Autodesk Inventor part; units mm, degrees
(part 2 of 3)
sketch "スケッチ2" plane through (0, 0, 3) normal (0, 0, 1) x (1, 0, 0)
  line L0 (168.378, 87.7618) -> (167.765, 88.2934) projected
  arc A0 (167.765, 88.2934) -> (169.0746, 89.9356) centre (148.5, 105) ccw projected
  line L1 (169.0746, 89.9356) -> (169.7292, 89.4562) projected
  arc A1 (169.7292, 89.4562) -> (170.0536, 89.2707) centre (171.1243, 91.5187) ccw projected
  arc A2 (170.0536, 89.2707) -> (171.1838, 88.8403) centre (173.0427, 95.4208) ccw projected
  arc A3 (171.1838, 88.8403) -> (173.5053, 88.4249) centre (174.4109, 100.1798) ccw projected
  arc A4 (173.5053, 88.4249) -> (174.2831, 89.6627) centre (148.5, 105) ccw projected
  arc A5 (174.2831, 89.6627) -> (172.9015, 91.5741) centre (164.0852, 83.7465) ccw projected
  arc A6 (172.9015, 91.5741) -> (172.0234, 92.4056) centre (167.7792, 87.0441) ccw projected
  arc A7 (172.0234, 92.4056) -> (171.7155, 92.6173) centre (170.4625, 90.4655) ccw projected
  line L2 (171.7155, 92.6173) -> (170.9996, 92.9992) projected
  arc A8 (170.9996, 92.9992) -> (171.9109, 94.8915) centre (148.5, 105) ccw projected
  line L3 (171.9109, 94.8915) -> (172.6558, 94.5699) projected
  arc A9 (172.6558, 94.5699) -> (173.0133, 94.4612) centre (173.5569, 96.8911) ccw projected
  arc A10 (173.0133, 94.4612) -> (174.2109, 94.2931) centre (174.5589, 101.1222) ccw projected
  arc A11 (174.2109, 94.2931) -> (176.5667, 94.4046) centre (174.8339, 106.0664) ccw projected
  arc A12 (176.5667, 94.4046) -> (177.0495, 95.7845) centre (148.5, 105) ccw projected
  arc A13 (177.0495, 95.7845) -> (175.2773, 97.3405) centre (168.4238, 87.7474) ccw projected
  arc A14 (175.2773, 97.3405) -> (174.2362, 97.9558) centre (171.2914, 91.7843) ccw projected
  arc A15 (174.2362, 97.9558) -> (173.8888, 98.0937) centre (173.1461, 95.717) ccw projected
  line L4 (173.8888, 98.0937) -> (173.1059, 98.3067) projected
  arc A16 (173.1059, 98.3067) -> (173.5733, 100.3544) centre (148.5, 105) ccw projected
  line L5 (173.5733, 100.3544) -> (174.3711, 100.2066) projected
  arc A17 (174.3711, 100.2066) -> (174.7439, 100.1801) centre (174.7331, 102.6701) ccw projected
  arc A18 (174.7439, 100.1801) -> (175.9488, 100.2827) centre (174.7684, 107.0181) ccw projected
  arc A19 (175.9488, 100.2827) -> (178.2207, 100.9157) centre (173.9363, 111.8995) ccw projected
  arc A20 (178.2207, 100.9157) -> (178.3844, 102.3684) centre (148.5, 105) ccw projected
  arc A21 (178.3844, 102.3684) -> (176.3103, 103.4911) centre (171.7633, 92.6134) ccw projected
  arc A22 (176.3103, 103.4911) -> (175.1584, 103.8592) centre (173.6608, 97.1872) ccw projected
  arc A23 (175.1584, 103.8592) -> (174.7891, 103.9164) centre (174.5938, 101.4341) ccw projected
  line L6 (174.7891, 103.9164) -> (173.9784, 103.9498) projected
  arc A24 (173.9784, 103.9498) -> (173.9784, 106.0502) centre (148.5, 105) ccw projected
  line L7 (173.9784, 106.0502) -> (174.7891, 106.0836) projected
  arc A25 (174.7891, 106.0836) -> (175.1584, 106.1408) centre (174.5938, 108.5659) ccw projected
  arc A26 (175.1584, 106.1408) -> (176.3103, 106.5089) centre (173.6608, 112.8128) ccw projected
  arc A27 (176.3103, 106.5089) -> (178.3844, 107.6316) centre (171.7633, 117.3866) ccw projected
  arc A28 (178.3844, 107.6316) -> (178.2207, 109.0843) centre (148.5, 105) ccw projected
  arc A29 (178.2207, 109.0843) -> (175.9488, 109.7173) centre (173.9363, 98.1005) ccw projected
  arc A30 (175.9488, 109.7173) -> (174.7439, 109.8199) centre (174.7684, 102.9819) ccw projected
  arc A31 (174.7439, 109.8199) -> (174.3711, 109.7934) centre (174.7331, 107.3299) ccw projected
  line L8 (174.3711, 109.7934) -> (173.5733, 109.6456) projected
  arc A32 (173.5733, 109.6456) -> (173.1059, 111.6933) centre (148.5, 105) ccw projected
  line L9 (173.1059, 111.6933) -> (173.8888, 111.9063) projected
  arc A33 (173.8888, 111.9063) -> (174.2362, 112.0442) centre (173.1461, 114.283) ccw projected
  arc A34 (174.2362, 112.0442) -> (175.2773, 112.6595) centre (171.2914, 118.2157) ccw projected
  arc A35 (175.2773, 112.6595) -> (177.0495, 114.2155) centre (168.4238, 122.2526) ccw projected
  arc A36 (177.0495, 114.2155) -> (176.5667, 115.5954) centre (148.5, 105) ccw projected
  arc A37 (176.5667, 115.5954) -> (174.2109, 115.7069) centre (174.8339, 103.9336) ccw projected
  arc A38 (174.2109, 115.7069) -> (173.0133, 115.5388) centre (174.5589, 108.8778) ccw projected
  arc A39 (173.0133, 115.5388) -> (172.6558, 115.4301) centre (173.5569, 113.1089) ccw projected
  line L10 (172.6558, 115.4301) -> (171.9109, 115.1085) projected
  arc A40 (171.9109, 115.1085) -> (170.9996, 117.0008) centre (148.5, 105) ccw projected
  line L11 (170.9996, 117.0008) -> (171.7155, 117.3827) projected
  arc A41 (171.7155, 117.3827) -> (172.0234, 117.5944) centre (170.4625, 119.5345) ccw projected
  arc A42 (172.0234, 117.5944) -> (172.9015, 118.4259) centre (167.7792, 122.9559) ccw projected
  arc A43 (172.9015, 118.4259) -> (174.2831, 120.3373) centre (164.0852, 126.2535) ccw projected
  arc A44 (174.2831, 120.3373) -> (173.5053, 121.5751) centre (148.5, 105) ccw projected
  arc A45 (173.5053, 121.5751) -> (171.1838, 121.1597) centre (174.4109, 109.8202) ccw projected
  arc A46 (171.1838, 121.1597) -> (170.0536, 120.7293) centre (173.0427, 114.5792) ccw projected
  arc A47 (170.0536, 120.7293) -> (169.7292, 120.5438) centre (171.1243, 118.4813) ccw projected
  line L12 (169.7292, 120.5438) -> (169.0746, 120.0644) projected
  arc A48 (169.0746, 120.0644) -> (167.765, 121.7066) centre (148.5, 105) ccw projected
  line L13 (167.765, 121.7066) -> (168.378, 122.2382) projected
  arc A49 (168.378, 122.2382) -> (168.6311, 122.5131) centre (166.6776, 124.0572) ccw projected
  arc A50 (168.6311, 122.5131) -> (169.3022, 123.5192) centre (163.3003, 126.7958) ccw projected
  arc A51 (169.3022, 123.5192) -> (170.2238, 125.69) centre (158.9651, 129.1887) ccw projected
  arc A52 (170.2238, 125.69) -> (169.19, 126.7238) centre (148.5, 105) ccw projected
  arc A53 (169.19, 126.7238) -> (167.0192, 125.8022) centre (172.6887, 115.4651) ccw projected
  arc A54 (167.0192, 125.8022) -> (166.0131, 125.1311) centre (170.2958, 119.8003) ccw projected
  arc A55 (166.0131, 125.1311) -> (165.7382, 124.878) centre (167.5572, 123.1776) ccw projected
  line L14 (165.7382, 124.878) -> (165.2066, 124.265) projected
  arc A56 (165.2066, 124.265) -> (163.5644, 125.5746) centre (148.5, 105) ccw projected
  line L15 (163.5644, 125.5746) -> (164.0438, 126.2292) projected
  arc A57 (164.0438, 126.2292) -> (164.2293, 126.5536) centre (161.9813, 127.6243) ccw projected
  arc A58 (164.2293, 126.5536) -> (164.6597, 127.6838) centre (158.0792, 129.5427) ccw projected
  arc A59 (164.6597, 127.6838) -> (165.0751, 130.0053) centre (153.3202, 130.9109) ccw projected
  arc A60 (165.0751, 130.0053) -> (163.8373, 130.7831) centre (148.5, 105) ccw projected
  arc A61 (163.8373, 130.7831) -> (161.9259, 129.4015) centre (169.7535, 120.5852) ccw projected
  arc A62 (161.9259, 129.4015) -> (161.0944, 128.5234) centre (166.4559, 124.2792) ccw projected
  arc A63 (161.0944, 128.5234) -> (160.8827, 128.2155) centre (163.0345, 126.9625) ccw projected
  line L16 (160.8827, 128.2155) -> (160.5008, 127.4996) projected
  arc A64 (160.5008, 127.4996) -> (158.6085, 128.4109) centre (148.5, 105) ccw projected
  line L17 (158.6085, 128.4109) -> (158.9301, 129.1558) projected
  arc A65 (158.9301, 129.1558) -> (159.0388, 129.5133) centre (156.6089, 130.0569) ccw projected
  arc A66 (159.0388, 129.5133) -> (159.2069, 130.7109) centre (152.3778, 131.0589) ccw projected
  arc A67 (159.2069, 130.7109) -> (159.0954, 133.0667) centre (147.4336, 131.3339) ccw projected
  arc A68 (159.0954, 133.0667) -> (157.7155, 133.5495) centre (148.5, 105) ccw projected
  arc A69 (157.7155, 133.5495) -> (156.1595, 131.7773) centre (165.7526, 124.9238) ccw projected
  arc A70 (156.1595, 131.7773) -> (155.5442, 130.7362) centre (161.7157, 127.7914) ccw projected
  arc A71 (155.5442, 130.7362) -> (155.4063, 130.3888) centre (157.783, 129.6461) ccw projected
  line L18 (155.4063, 130.3888) -> (155.1933, 129.6059) projected
  arc A72 (155.1933, 129.6059) -> (153.1456, 130.0733) centre (148.5, 105) ccw projected
  line L19 (153.1456, 130.0733) -> (153.2934, 130.8711) projected
  arc A73 (153.2934, 130.8711) -> (153.3199, 131.2439) centre (150.8299, 131.2331) ccw projected
  arc A74 (153.3199, 131.2439) -> (153.2173, 132.4488) centre (146.4819, 131.2684) ccw projected
  arc A75 (153.2173, 132.4488) -> (152.5843, 134.7207) centre (141.6005, 130.4363) ccw projected
  arc A76 (152.5843, 134.7207) -> (151.1316, 134.8844) centre (148.5, 105) ccw projected
  arc A77 (151.1316, 134.8844) -> (150.0089, 132.8103) centre (160.8866, 128.2633) ccw projected
  arc A78 (150.0089, 132.8103) -> (149.6408, 131.6584) centre (156.3128, 130.1608) ccw projected
  arc A79 (149.6408, 131.6584) -> (149.5836, 131.2891) centre (152.0659, 131.0938) ccw projected
  line L20 (149.5836, 131.2891) -> (149.5502, 130.4784) projected
  arc A80 (149.5502, 130.4784) -> (147.4498, 130.4784) centre (148.5, 105) ccw projected
  line L21 (147.4498, 130.4784) -> (147.4164, 131.2891) projected
  arc A81 (147.4164, 131.2891) -> (147.3592, 131.6584) centre (144.9341, 131.0938) ccw projected
  arc A82 (147.3592, 131.6584) -> (146.9911, 132.8103) centre (140.6872, 130.1608) ccw projected
  arc A83 (146.9911, 132.8103) -> (145.8684, 134.8844) centre (136.1134, 128.2633) ccw projected
  arc A84 (145.8684, 134.8844) -> (144.4157, 134.7207) centre (148.5, 105) ccw projected
  arc A85 (144.4157, 134.7207) -> (143.7827, 132.4488) centre (155.3995, 130.4363) ccw projected
  arc A86 (143.7827, 132.4488) -> (143.6801, 131.2439) centre (150.5181, 131.2684) ccw projected
  arc A87 (143.6801, 131.2439) -> (143.7066, 130.8711) centre (146.1701, 131.2331) ccw projected
  line L22 (143.7066, 130.8711) -> (143.8544, 130.0733) projected
  arc A88 (143.8544, 130.0733) -> (141.8067, 129.6059) centre (148.5, 105) ccw projected
  line L23 (141.8067, 129.6059) -> (141.5937, 130.3888) projected
  arc A89 (141.5937, 130.3888) -> (141.4558, 130.7362) centre (139.217, 129.6461) ccw projected
  arc A90 (141.4558, 130.7362) -> (140.8405, 131.7773) centre (135.2843, 127.7914) ccw projected
  arc A91 (140.8405, 131.7773) -> (139.2845, 133.5495) centre (131.2474, 124.9238) ccw projected
  arc A92 (139.2845, 133.5495) -> (137.9046, 133.0667) centre (148.5, 105) ccw projected
  arc A93 (137.9046, 133.0667) -> (137.7931, 130.7109) centre (149.5664, 131.3339) ccw projected
  arc A94 (137.7931, 130.7109) -> (137.9612, 129.5133) centre (144.6222, 131.0589) ccw projected
  arc A95 (137.9612, 129.5133) -> (138.0699, 129.1558) centre (140.3911, 130.0569) ccw projected
  line L24 (138.0699, 129.1558) -> (138.3915, 128.4109) projected
  arc A96 (138.3915, 128.4109) -> (136.4992, 127.4996) centre (148.5, 105) ccw projected
  line L25 (136.4992, 127.4996) -> (136.1173, 128.2155) projected
  arc A97 (136.1173, 128.2155) -> (135.9056, 128.5234) centre (133.9655, 126.9625) ccw projected
  arc A98 (135.9056, 128.5234) -> (135.0741, 129.4015) centre (130.5441, 124.2792) ccw projected
  arc A99 (135.0741, 129.4015) -> (133.1627, 130.7831) centre (127.2465, 120.5852) ccw projected
  arc A100 (133.1627, 130.7831) -> (131.9249, 130.0053) centre (148.5, 105) ccw projected
  arc A101 (131.9249, 130.0053) -> (132.3403, 127.6838) centre (143.6798, 130.9109) ccw projected
  arc A102 (132.3403, 127.6838) -> (132.7707, 126.5536) centre (138.9208, 129.5427) ccw projected
  arc A103 (132.7707, 126.5536) -> (132.9562, 126.2292) centre (135.0187, 127.6243) ccw projected
  line L26 (132.9562, 126.2292) -> (133.4356, 125.5746) projected
  arc A104 (133.4356, 125.5746) -> (131.7934, 124.265) centre (148.5, 105) ccw projected
  line L27 (131.7934, 124.265) -> (131.2618, 124.878) projected
  arc A105 (131.2618, 124.878) -> (130.9869, 125.1311) centre (129.4428, 123.1776) ccw projected
  arc A106 (130.9869, 125.1311) -> (129.9808, 125.8022) centre (126.7042, 119.8003) ccw projected
  arc A107 (129.9808, 125.8022) -> (127.81, 126.7238) centre (124.3113, 115.4651) ccw projected
  arc A108 (127.81, 126.7238) -> (126.7762, 125.69) centre (148.5, 105) ccw projected
  arc A109 (126.7762, 125.69) -> (127.6978, 123.5192) centre (138.0349, 129.1887) ccw projected
  arc A110 (127.6978, 123.5192) -> (128.3689, 122.5131) centre (133.6997, 126.7958) ccw projected
  arc A111 (128.3689, 122.5131) -> (128.622, 122.2382) centre (130.3224, 124.0572) ccw projected
  line L28 (128.622, 122.2382) -> (129.235, 121.7066) projected
  arc A112 (129.235, 121.7066) -> (127.9254, 120.0644) centre (148.5, 105) ccw projected
  line L29 (127.9254, 120.0644) -> (127.2708, 120.5438) projected
  arc A113 (127.2708, 120.5438) -> (126.9464, 120.7293) centre (125.8757, 118.4813) ccw projected
  arc A114 (126.9464, 120.7293) -> (125.8162, 121.1597) centre (123.9573, 114.5792) ccw projected
  arc A115 (125.8162, 121.1597) -> (123.4947, 121.5751) centre (122.5891, 109.8202) ccw projected
  arc A116 (123.4947, 121.5751) -> (122.7169, 120.3373) centre (148.5, 105) ccw projected
  arc A117 (122.7169, 120.3373) -> (124.0985, 118.4259) centre (132.9148, 126.2535) ccw projected
  arc A118 (124.0985, 118.4259) -> (124.9766, 117.5944) centre (129.2208, 122.9559) ccw projected
  arc A119 (124.9766, 117.5944) -> (125.2845, 117.3827) centre (126.5375, 119.5345) ccw projected
  line L30 (125.2845, 117.3827) -> (126.0004, 117.0008) projected
  arc A120 (126.0004, 117.0008) -> (125.0891, 115.1085) centre (148.5, 105) ccw projected
  line L31 (125.0891, 115.1085) -> (124.3442, 115.4301) projected
  arc A121 (124.3442, 115.4301) -> (123.9867, 115.5388) centre (123.4431, 113.1089) ccw projected
  arc A122 (123.9867, 115.5388) -> (122.7891, 115.7069) centre (122.4411, 108.8778) ccw projected
  arc A123 (122.7891, 115.7069) -> (120.4333, 115.5954) centre (122.1661, 103.9336) ccw projected
  arc A124 (120.4333, 115.5954) -> (119.9505, 114.2155) centre (148.5, 105) ccw projected
  arc A125 (119.9505, 114.2155) -> (121.7227, 112.6595) centre (128.5762, 122.2526) ccw projected
  arc A126 (121.7227, 112.6595) -> (122.7638, 112.0442) centre (125.7086, 118.2157) ccw projected
  arc A127 (122.7638, 112.0442) -> (123.1112, 111.9063) centre (123.8539, 114.283) ccw projected
  line L32 (123.1112, 111.9063) -> (123.8941, 111.6933) projected
  arc A128 (123.8941, 111.6933) -> (123.4267, 109.6456) centre (148.5, 105) ccw projected
  line L33 (123.4267, 109.6456) -> (122.6289, 109.7934) projected
  arc A129 (122.6289, 109.7934) -> (122.2561, 109.8199) centre (122.2669, 107.3299) ccw projected
  arc A130 (122.2561, 109.8199) -> (121.0512, 109.7173) centre (122.2316, 102.9819) ccw projected
  arc A131 (121.0512, 109.7173) -> (118.7793, 109.0843) centre (123.0637, 98.1005) ccw projected
  arc A132 (118.7793, 109.0843) -> (118.6156, 107.6316) centre (148.5, 105) ccw projected
  arc A133 (118.6156, 107.6316) -> (120.6897, 106.5089) centre (125.2367, 117.3866) ccw projected
  arc A134 (120.6897, 106.5089) -> (121.8416, 106.1408) centre (123.3392, 112.8128) ccw projected
  arc A135 (121.8416, 106.1408) -> (122.2109, 106.0836) centre (122.4062, 108.5659) ccw projected
  line L34 (122.2109, 106.0836) -> (123.0216, 106.0502) projected
  arc A136 (123.0216, 106.0502) -> (123.0216, 103.9498) centre (148.5, 105) ccw projected
  line L35 (123.0216, 103.9498) -> (122.2109, 103.9164) projected
  arc A137 (122.2109, 103.9164) -> (121.8416, 103.8592) centre (122.4062, 101.4341) ccw projected
  arc A138 (121.8416, 103.8592) -> (120.6897, 103.4911) centre (123.3392, 97.1872) ccw projected
  arc A139 (120.6897, 103.4911) -> (118.6156, 102.3684) centre (125.2367, 92.6134) ccw projected
  arc A140 (118.6156, 102.3684) -> (118.7793, 100.9157) centre (148.5, 105) ccw projected
  arc A141 (118.7793, 100.9157) -> (121.0512, 100.2827) centre (123.0637, 111.8995) ccw projected
  arc A142 (121.0512, 100.2827) -> (122.2561, 100.1801) centre (122.2316, 107.0181) ccw projected
  arc A143 (122.2561, 100.1801) -> (122.6289, 100.2066) centre (122.2669, 102.6701) ccw projected
  line L36 (122.6289, 100.2066) -> (123.4267, 100.3544) projected
  arc A144 (123.4267, 100.3544) -> (123.8941, 98.3067) centre (148.5, 105) ccw projected
  line L37 (123.8941, 98.3067) -> (123.1112, 98.0937) projected
  arc A145 (123.1112, 98.0937) -> (122.7638, 97.9558) centre (123.8539, 95.717) ccw projected
  arc A146 (122.7638, 97.9558) -> (121.7227, 97.3405) centre (125.7086, 91.7843) ccw projected
  arc A147 (121.7227, 97.3405) -> (119.9505, 95.7845) centre (128.5762, 87.7474) ccw projected
  arc A148 (119.9505, 95.7845) -> (120.4333, 94.4046) centre (148.5, 105) ccw projected
  arc A149 (120.4333, 94.4046) -> (122.7891, 94.2931) centre (122.1661, 106.0664) ccw projected
  arc A150 (122.7891, 94.2931) -> (123.9867, 94.4612) centre (122.4411, 101.1222) ccw projected
  arc A151 (123.9867, 94.4612) -> (124.3442, 94.5699) centre (123.4431, 96.8911) ccw projected
  line L38 (124.3442, 94.5699) -> (125.0891, 94.8915) projected
  arc A152 (125.0891, 94.8915) -> (126.0004, 92.9992) centre (148.5, 105) ccw projected
  line L39 (126.0004, 92.9992) -> (125.2845, 92.6173) projected
  arc A153 (125.2845, 92.6173) -> (124.9766, 92.4056) centre (126.5375, 90.4655) ccw projected
  arc A154 (124.9766, 92.4056) -> (124.0985, 91.5741) centre (129.2208, 87.0441) ccw projected
  arc A155 (124.0985, 91.5741) -> (122.7169, 89.6627) centre (132.9148, 83.7465) ccw projected
  arc A156 (122.7169, 89.6627) -> (123.4947, 88.4249) centre (148.5, 105) ccw projected
  arc A157 (123.4947, 88.4249) -> (125.8162, 88.8403) centre (122.5891, 100.1798) ccw projected
  arc A158 (125.8162, 88.8403) -> (126.9464, 89.2707) centre (123.9573, 95.4208) ccw projected
  arc A159 (126.9464, 89.2707) -> (127.2708, 89.4562) centre (125.8757, 91.5187) ccw projected
  line L40 (127.2708, 89.4562) -> (127.9254, 89.9356) projected
  arc A160 (127.9254, 89.9356) -> (129.235, 88.2934) centre (148.5, 105) ccw projected
  line L41 (129.235, 88.2934) -> (128.622, 87.7618) projected
  arc A161 (128.622, 87.7618) -> (128.3689, 87.4869) centre (130.3224, 85.9428) ccw projected
  arc A162 (128.3689, 87.4869) -> (127.6978, 86.4808) centre (133.6997, 83.2042) ccw projected
  arc A163 (127.6978, 86.4808) -> (126.7762, 84.31) centre (138.0349, 80.8113) ccw projected
  arc A164 (126.7762, 84.31) -> (127.81, 83.2762) centre (148.5, 105) ccw projected
  arc A165 (127.81, 83.2762) -> (129.9808, 84.1978) centre (124.3113, 94.5349) ccw projected
  arc A166 (129.9808, 84.1978) -> (130.9869, 84.8689) centre (126.7042, 90.1997) ccw projected
  arc A167 (130.9869, 84.8689) -> (131.2618, 85.122) centre (129.4428, 86.8224) ccw projected
  line L42 (131.2618, 85.122) -> (131.7934, 85.735) projected
  arc A168 (131.7934, 85.735) -> (133.4356, 84.4254) centre (148.5, 105) ccw projected
  line L43 (133.4356, 84.4254) -> (132.9562, 83.7708) projected
  arc A169 (132.9562, 83.7708) -> (132.7707, 83.4464) centre (135.0187, 82.3757) ccw projected
  arc A170 (132.7707, 83.4464) -> (132.3403, 82.3162) centre (138.9208, 80.4573) ccw projected
  arc A171 (132.3403, 82.3162) -> (131.9249, 79.9947) centre (143.6798, 79.0891) ccw projected
  arc A172 (131.9249, 79.9947) -> (133.1627, 79.2169) centre (148.5, 105) ccw projected
  arc A173 (133.1627, 79.2169) -> (135.0741, 80.5985) centre (127.2465, 89.4148) ccw projected
  arc A174 (135.0741, 80.5985) -> (135.9056, 81.4766) centre (130.5441, 85.7208) ccw projected
  arc A175 (135.9056, 81.4766) -> (136.1173, 81.7845) centre (133.9655, 83.0375) ccw projected
  line L44 (136.1173, 81.7845) -> (136.4992, 82.5004) projected
  arc A176 (136.4992, 82.5004) -> (138.3915, 81.5891) centre (148.5, 105) ccw projected
  line L45 (138.3915, 81.5891) -> (138.0699, 80.8442) projected
  arc A177 (138.0699, 80.8442) -> (137.9612, 80.4867) centre (140.3911, 79.9431) ccw projected
  arc A178 (137.9612, 80.4867) -> (137.7931, 79.2891) centre (144.6222, 78.9411) ccw projected
  arc A179 (137.7931, 79.2891) -> (137.9046, 76.9333) centre (149.5664, 78.6661) ccw projected
  arc A180 (137.9046, 76.9333) -> (139.2845, 76.4505) centre (148.5, 105) ccw projected
  arc A181 (139.2845, 76.4505) -> (140.8405, 78.2227) centre (131.2474, 85.0762) ccw projected
  arc A182 (140.8405, 78.2227) -> (141.4558, 79.2638) centre (135.2843, 82.2086) ccw projected
  arc A183 (141.4558, 79.2638) -> (141.5937, 79.6112) centre (139.217, 80.3539) ccw projected
  line L46 (141.5937, 79.6112) -> (141.8067, 80.3941) projected
  arc A184 (141.8067, 80.3941) -> (143.8544, 79.9267) centre (148.5, 105) ccw projected
  line L47 (143.8544, 79.9267) -> (143.7066, 79.1289) projected
  arc A185 (143.7066, 79.1289) -> (143.6801, 78.7561) centre (146.1701, 78.7669) ccw projected
  arc A186 (143.6801, 78.7561) -> (143.7827, 77.5512) centre (150.5181, 78.7316) ccw projected
  arc A187 (143.7827, 77.5512) -> (144.4157, 75.2793) centre (155.3995, 79.5637) ccw projected
  arc A188 (144.4157, 75.2793) -> (145.8684, 75.1156) centre (148.5, 105) ccw projected
  arc A189 (145.8684, 75.1156) -> (146.9911, 77.1897) centre (136.1134, 81.7367) ccw projected
  arc A190 (146.9911, 77.1897) -> (147.3592, 78.3416) centre (140.6872, 79.8392) ccw projected
  arc A191 (147.3592, 78.3416) -> (147.4164, 78.7109) centre (144.9341, 78.9062) ccw projected
  line L48 (147.4164, 78.7109) -> (147.4498, 79.5216) projected
  arc A192 (147.4498, 79.5216) -> (149.5502, 79.5216) centre (148.5, 105) ccw projected
  line L49 (149.5502, 79.5216) -> (149.5836, 78.7109) projected
  arc A193 (149.5836, 78.7109) -> (149.6408, 78.3416) centre (152.0659, 78.9062) ccw projected
  arc A194 (149.6408, 78.3416) -> (150.0089, 77.1897) centre (156.3128, 79.8392) ccw projected
  arc A195 (150.0089, 77.1897) -> (151.1316, 75.1156) centre (160.8866, 81.7367) ccw projected
  arc A196 (151.1316, 75.1156) -> (152.5843, 75.2793) centre (148.5, 105) ccw projected
  arc A197 (152.5843, 75.2793) -> (153.2173, 77.5512) centre (141.6005, 79.5637) ccw projected
  arc A198 (153.2173, 77.5512) -> (153.3199, 78.7561) centre (146.4819, 78.7316) ccw projected
  arc A199 (153.3199, 78.7561) -> (153.2934, 79.1289) centre (150.8299, 78.7669) ccw projected
  line L50 (153.2934, 79.1289) -> (153.1456, 79.9267) projected
  arc A200 (153.1456, 79.9267) -> (155.1933, 80.3941) centre (148.5, 105) ccw projected
  line L51 (155.1933, 80.3941) -> (155.4063, 79.6112) projected
  arc A201 (155.4063, 79.6112) -> (155.5442, 79.2638) centre (157.783, 80.3539) ccw projected
  arc A202 (155.5442, 79.2638) -> (156.1595, 78.2227) centre (161.7157, 82.2086) ccw projected
  arc A203 (156.1595, 78.2227) -> (157.7155, 76.4505) centre (165.7526, 85.0762) ccw projected
  arc A204 (157.7155, 76.4505) -> (159.0954, 76.9333) centre (148.5, 105) ccw projected
  arc A205 (159.0954, 76.9333) -> (159.2069, 79.2891) centre (147.4336, 78.6661) ccw projected
  arc A206 (159.2069, 79.2891) -> (159.0388, 80.4867) centre (152.3778, 78.9411) ccw projected
  arc A207 (159.0388, 80.4867) -> (158.9301, 80.8442) centre (156.6089, 79.9431) ccw projected
  line L52 (158.9301, 80.8442) -> (158.6085, 81.5891) projected
  arc A208 (158.6085, 81.5891) -> (160.5008, 82.5004) centre (148.5, 105) ccw projected
  line L53 (160.5008, 82.5004) -> (160.8827, 81.7845) projected
  arc A209 (160.8827, 81.7845) -> (161.0944, 81.4766) centre (163.0345, 83.0375) ccw projected
  arc A210 (161.0944, 81.4766) -> (161.9259, 80.5985) centre (166.4559, 85.7208) ccw projected
  arc A211 (161.9259, 80.5985) -> (163.8373, 79.2169) centre (169.7535, 89.4148) ccw projected
  arc A212 (163.8373, 79.2169) -> (165.0751, 79.9947) centre (148.5, 105) ccw projected
  arc A213 (165.0751, 79.9947) -> (164.6597, 82.3162) centre (153.3202, 79.0891) ccw projected
  arc A214 (164.6597, 82.3162) -> (164.2293, 83.4464) centre (158.0792, 80.4573) ccw projected
  arc A215 (164.2293, 83.4464) -> (164.0438, 83.7708) centre (161.9813, 82.3757) ccw projected
  line L54 (164.0438, 83.7708) -> (163.5644, 84.4254) projected
  arc A216 (163.5644, 84.4254) -> (165.2066, 85.735) centre (148.5, 105) ccw projected
  line L55 (165.2066, 85.735) -> (165.7382, 85.122) projected
  arc A217 (165.7382, 85.122) -> (166.0131, 84.8689) centre (167.5572, 86.8224) ccw projected
  arc A218 (166.0131, 84.8689) -> (167.0192, 84.1978) centre (170.2958, 90.1997) ccw projected
  arc A219 (167.0192, 84.1978) -> (169.19, 83.2762) centre (172.6887, 94.5349) ccw projected
  arc A220 (169.19, 83.2762) -> (170.2238, 84.31) centre (148.5, 105) ccw projected
  arc A221 (170.2238, 84.31) -> (169.3022, 86.4808) centre (158.9651, 80.8113) ccw projected
  arc A222 (169.3022, 86.4808) -> (168.6311, 87.4869) centre (163.3003, 83.2042) ccw projected
  arc A223 (168.6311, 87.4869) -> (168.378, 87.7618) centre (166.6776, 85.9428) ccw projected
  arc A224 (148.5, 98.8449) -> (147.3388, 98.1857) centre (148.8502, 96.8758) ccw projected
  arc A225 (148.5, 98.8449) -> (148.2359, 98.874) centre (148.1498, 96.8758) ccw projected
  arc A226 (148.2359, 98.874) -> (148.7641, 98.874) centre (148.5, 105) ccw projected
  arc A227 (148.7641, 98.874) -> (148.5, 98.8449) centre (148.8502, 96.8758) ccw projected
  arc A228 (149.6612, 98.1857) -> (148.5, 98.8449) centre (148.1498, 96.8758) ccw projected
  line L56 (149.6612, 98.1857) -> (158.7085, 87.7462) projected
  arc A229 (158.0456, 84.6252) -> (158.7085, 87.7462) centre (157.1971, 86.4363) ccw projected
  arc A230 (138.9544, 84.6252) -> (158.0456, 84.6252) centre (148.5, 105) ccw projected
  arc A231 (138.2915, 87.7462) -> (138.9544, 84.6252) centre (139.8029, 86.4363) ccw projected
  line L57 (138.2915, 87.7462) -> (147.3388, 98.1857) projected
  arc A232 (154.3538, 103.098) -> (154.622, 101.7899) centre (156.3348, 102.8226) ccw projected
  arc A233 (154.3538, 103.098) -> (154.2446, 102.8558) centre (156.1183, 102.1564) ccw projected
  arc A234 (154.2446, 102.8558) -> (154.4078, 103.3581) centre (148.5, 105) ccw projected
  arc A235 (154.4078, 103.3581) -> (154.3538, 103.098) centre (156.3348, 102.8226) ccw projected
  arc A236 (155.3396, 103.9986) -> (154.3538, 103.098) centre (156.1183, 102.1564) ccw projected
  line L58 (155.3396, 103.9986) -> (168.064, 109.3772) projected
  arc A237 (170.8273, 107.7823) -> (168.064, 109.3772) centre (168.8427, 107.535) ccw projected
  arc A238 (164.9278, 89.6254) -> (170.8273, 107.7823) centre (148.5, 105) ccw projected
  arc A239 (161.7547, 89.9594) -> (164.9278, 89.6254) centre (163.4675, 90.992) ccw projected
  line L59 (161.7547, 89.9594) -> (154.622, 101.7899) projected
  arc A240 (142.7554, 102.8558) -> (142.6462, 103.098) centre (140.8817, 102.1564) ccw projected
  arc A241 (142.378, 101.7899) -> (142.6462, 103.098) centre (140.6652, 102.8226) ccw projected
  line L60 (142.378, 101.7899) -> (135.2453, 89.9594) projected
  arc A242 (132.0722, 89.6254) -> (135.2453, 89.9594) centre (133.5325, 90.992) ccw projected
  arc A243 (126.1727, 107.7823) -> (132.0722, 89.6254) centre (148.5, 105) ccw projected
  arc A244 (128.936, 109.3772) -> (126.1727, 107.7823) centre (128.1573, 107.535) ccw projected
  line L61 (128.936, 109.3772) -> (141.6604, 103.9986) projected
  arc A245 (142.6462, 103.098) -> (141.6604, 103.9986) centre (140.8817, 102.1564) ccw projected
  arc A246 (142.6462, 103.098) -> (142.5922, 103.3581) centre (140.6652, 102.8226) ccw projected
  arc A247 (142.5922, 103.3581) -> (142.7554, 102.8558) centre (148.5, 105) ccw projected
  line L62 (166.9004, 112.9582) -> (153.4448, 109.8304) projected
  arc A248 (152.1179, 109.9796) -> (153.4448, 109.8304) centre (152.9919, 111.7784) ccw projected
  arc A249 (151.566, 111.1954) -> (152.1179, 109.9796) centre (153.5586, 111.3667) ccw projected
  line L63 (151.566, 111.1954) -> (150.3827, 124.9591) projected
  arc A250 (152.7534, 127.0943) -> (150.3827, 124.9591) centre (152.3753, 125.1304) ccw projected
  arc A251 (168.1986, 115.8727) -> (152.7534, 127.0943) centre (148.5, 105) ccw projected
  arc A252 (166.9004, 112.9582) -> (168.1986, 115.8727) centre (166.4476, 114.9063) ccw projected
  arc A253 (144.8821, 109.9796) -> (145.434, 111.1954) centre (143.4414, 111.3667) ccw projected
  arc A254 (143.5552, 109.8304) -> (144.8821, 109.9796) centre (144.0081, 111.7784) ccw projected
  line L64 (143.5552, 109.8304) -> (130.0996, 112.9582) projected
  arc A255 (128.8014, 115.8727) -> (130.0996, 112.9582) centre (130.5524, 114.9063) ccw projected
  arc A256 (144.2466, 127.0943) -> (128.8014, 115.8727) centre (148.5, 105) ccw projected
  arc A257 (146.6173, 124.9591) -> (144.2466, 127.0943) centre (144.6247, 125.1304) ccw projected
  line L65 (146.6173, 124.9591) -> (145.434, 111.1954) projected
  point P0 (0, 0)
sketch "スケッチ3" plane through (0, 0, 0) normal (0, 0, -1) x (-1, 0, 0)
  line L0 (-168.378, 87.7618) -> (-167.765, 88.2934) projected
  arc A0 (-168.378, 87.7618) -> (-168.6311, 87.4869) centre (-166.6776, 85.9428) ccw projected
  arc A1 (-168.6311, 87.4869) -> (-169.3022, 86.4808) centre (-163.3003, 83.2042) ccw projected
  arc A2 (-169.3022, 86.4808) -> (-170.2238, 84.31) centre (-158.9651, 80.8113) ccw projected
  arc A3 (-170.2238, 84.31) -> (-169.19, 83.2762) centre (-148.5, 105) ccw projected
  arc A4 (-169.19, 83.2762) -> (-167.0192, 84.1978) centre (-172.6887, 94.5349) ccw projected
  arc A5 (-167.0192, 84.1978) -> (-166.0131, 84.8689) centre (-170.2958, 90.1997) ccw projected
  arc A6 (-166.0131, 84.8689) -> (-165.7382, 85.122) centre (-167.5572, 86.8224) ccw projected
  line L1 (-165.2066, 85.735) -> (-165.7382, 85.122) projected
  arc A7 (-165.2066, 85.735) -> (-163.5644, 84.4254) centre (-148.5, 105) ccw projected
  line L2 (-164.0438, 83.7708) -> (-163.5644, 84.4254) projected
  arc A8 (-164.0438, 83.7708) -> (-164.2293, 83.4464) centre (-161.9813, 82.3757) ccw projected
  arc A9 (-164.2293, 83.4464) -> (-164.6597, 82.3162) centre (-158.0792, 80.4573) ccw projected
  arc A10 (-164.6597, 82.3162) -> (-165.0751, 79.9947) centre (-153.3202, 79.0891) ccw projected
  arc A11 (-165.0751, 79.9947) -> (-163.8373, 79.2169) centre (-148.5, 105) ccw projected
  arc A12 (-163.8373, 79.2169) -> (-161.9259, 80.5985) centre (-169.7535, 89.4148) ccw projected
  arc A13 (-161.9259, 80.5985) -> (-161.0944, 81.4766) centre (-166.4559, 85.7208) ccw projected
  arc A14 (-161.0944, 81.4766) -> (-160.8827, 81.7845) centre (-163.0345, 83.0375) ccw projected
  line L3 (-160.5008, 82.5004) -> (-160.8827, 81.7845) projected
  arc A15 (-160.5008, 82.5004) -> (-158.6085, 81.5891) centre (-148.5, 105) ccw projected
  line L4 (-158.9301, 80.8442) -> (-158.6085, 81.5891) projected
  arc A16 (-158.9301, 80.8442) -> (-159.0388, 80.4867) centre (-156.6089, 79.9431) ccw projected
  arc A17 (-159.0388, 80.4867) -> (-159.2069, 79.2891) centre (-152.3778, 78.9411) ccw projected
  arc A18 (-159.2069, 79.2891) -> (-159.0954, 76.9333) centre (-147.4336, 78.6661) ccw projected
  arc A19 (-159.0954, 76.9333) -> (-157.7155, 76.4505) centre (-148.5, 105) ccw projected
  arc A20 (-157.7155, 76.4505) -> (-156.1595, 78.2227) centre (-165.7526, 85.0762) ccw projected
  arc A21 (-156.1595, 78.2227) -> (-155.5442, 79.2638) centre (-161.7157, 82.2086) ccw projected
  arc A22 (-155.5442, 79.2638) -> (-155.4063, 79.6112) centre (-157.783, 80.3539) ccw projected
  line L5 (-155.1933, 80.3941) -> (-155.4063, 79.6112) projected
  arc A23 (-155.1933, 80.3941) -> (-153.1456, 79.9267) centre (-148.5, 105) ccw projected
  line L6 (-153.2934, 79.1289) -> (-153.1456, 79.9267) projected
  arc A24 (-153.2934, 79.1289) -> (-153.3199, 78.7561) centre (-150.8299, 78.7669) ccw projected
  arc A25 (-153.3199, 78.7561) -> (-153.2173, 77.5512) centre (-146.4819, 78.7316) ccw projected
  arc A26 (-153.2173, 77.5512) -> (-152.5843, 75.2793) centre (-141.6005, 79.5637) ccw projected
  arc A27 (-152.5843, 75.2793) -> (-151.1316, 75.1156) centre (-148.5, 105) ccw projected
  arc A28 (-151.1316, 75.1156) -> (-150.0089, 77.1897) centre (-160.8866, 81.7367) ccw projected
  arc A29 (-150.0089, 77.1897) -> (-149.6408, 78.3416) centre (-156.3128, 79.8392) ccw projected
  arc A30 (-149.6408, 78.3416) -> (-149.5836, 78.7109) centre (-152.0659, 78.9062) ccw projected
  line L7 (-149.5502, 79.5216) -> (-149.5836, 78.7109) projected
  arc A31 (-149.5502, 79.5216) -> (-147.4498, 79.5216) centre (-148.5, 105) ccw projected
  line L8 (-147.4164, 78.7109) -> (-147.4498, 79.5216) projected
  arc A32 (-147.4164, 78.7109) -> (-147.3592, 78.3416) centre (-144.9341, 78.9062) ccw projected
  arc A33 (-147.3592, 78.3416) -> (-146.9911, 77.1897) centre (-140.6872, 79.8392) ccw projected
  arc A34 (-146.9911, 77.1897) -> (-145.8684, 75.1156) centre (-136.1134, 81.7367) ccw projected
  arc A35 (-145.8684, 75.1156) -> (-144.4157, 75.2793) centre (-148.5, 105) ccw projected
  arc A36 (-144.4157, 75.2793) -> (-143.7827, 77.5512) centre (-155.3995, 79.5637) ccw projected
  arc A37 (-143.7827, 77.5512) -> (-143.6801, 78.7561) centre (-150.5181, 78.7316) ccw projected
  arc A38 (-143.6801, 78.7561) -> (-143.7066, 79.1289) centre (-146.1701, 78.7669) ccw projected
  line L9 (-143.8544, 79.9267) -> (-143.7066, 79.1289) projected
  arc A39 (-143.8544, 79.9267) -> (-141.8067, 80.3941) centre (-148.5, 105) ccw projected
  line L10 (-141.5937, 79.6112) -> (-141.8067, 80.3941) projected
  arc A40 (-141.5937, 79.6112) -> (-141.4558, 79.2638) centre (-139.217, 80.3539) ccw projected
  arc A41 (-141.4558, 79.2638) -> (-140.8405, 78.2227) centre (-135.2843, 82.2086) ccw projected
  arc A42 (-140.8405, 78.2227) -> (-139.2845, 76.4505) centre (-131.2474, 85.0762) ccw projected
  arc A43 (-139.2845, 76.4505) -> (-137.9046, 76.9333) centre (-148.5, 105) ccw projected
  arc A44 (-137.9046, 76.9333) -> (-137.7931, 79.2891) centre (-149.5664, 78.6661) ccw projected
  arc A45 (-137.7931, 79.2891) -> (-137.9612, 80.4867) centre (-144.6222, 78.9411) ccw projected
  arc A46 (-137.9612, 80.4867) -> (-138.0699, 80.8442) centre (-140.3911, 79.9431) ccw projected
  line L11 (-138.3915, 81.5891) -> (-138.0699, 80.8442) projected
  arc A47 (-138.3915, 81.5891) -> (-136.4992, 82.5004) centre (-148.5, 105) ccw projected
  line L12 (-136.1173, 81.7845) -> (-136.4992, 82.5004) projected
  arc A48 (-136.1173, 81.7845) -> (-135.9056, 81.4766) centre (-133.9655, 83.0375) ccw projected
  arc A49 (-135.9056, 81.4766) -> (-135.0741, 80.5985) centre (-130.5441, 85.7208) ccw projected
  arc A50 (-135.0741, 80.5985) -> (-133.1627, 79.2169) centre (-127.2465, 89.4148) ccw projected
  arc A51 (-133.1627, 79.2169) -> (-131.9249, 79.9947) centre (-148.5, 105) ccw projected
  arc A52 (-131.9249, 79.9947) -> (-132.3403, 82.3162) centre (-143.6798, 79.0891) ccw projected
  arc A53 (-132.3403, 82.3162) -> (-132.7707, 83.4464) centre (-138.9208, 80.4573) ccw projected
  arc A54 (-132.7707, 83.4464) -> (-132.9562, 83.7708) centre (-135.0187, 82.3757) ccw projected
  line L13 (-133.4356, 84.4254) -> (-132.9562, 83.7708) projected
  arc A55 (-133.4356, 84.4254) -> (-131.7934, 85.735) centre (-148.5, 105) ccw projected
  line L14 (-131.2618, 85.122) -> (-131.7934, 85.735) projected
  arc A56 (-131.2618, 85.122) -> (-130.9869, 84.8689) centre (-129.4428, 86.8224) ccw projected
  arc A57 (-130.9869, 84.8689) -> (-129.9808, 84.1978) centre (-126.7042, 90.1997) ccw projected
  arc A58 (-129.9808, 84.1978) -> (-127.81, 83.2762) centre (-124.3113, 94.5349) ccw projected
  arc A59 (-127.81, 83.2762) -> (-126.7762, 84.31) centre (-148.5, 105) ccw projected
  arc A60 (-126.7762, 84.31) -> (-127.6978, 86.4808) centre (-138.0349, 80.8113) ccw projected
  arc A61 (-127.6978, 86.4808) -> (-128.3689, 87.4869) centre (-133.6997, 83.2042) ccw projected
  arc A62 (-128.3689, 87.4869) -> (-128.622, 87.7618) centre (-130.3224, 85.9428) ccw projected
  line L15 (-129.235, 88.2934) -> (-128.622, 87.7618) projected
  arc A63 (-129.235, 88.2934) -> (-127.9254, 89.9356) centre (-148.5, 105) ccw projected
  line L16 (-127.2708, 89.4562) -> (-127.9254, 89.9356) projected
  arc A64 (-127.2708, 89.4562) -> (-126.9464, 89.2707) centre (-125.8757, 91.5187) ccw projected
  arc A65 (-126.9464, 89.2707) -> (-125.8162, 88.8403) centre (-123.9573, 95.4208) ccw projected
  arc A66 (-125.8162, 88.8403) -> (-123.4947, 88.4249) centre (-122.5891, 100.1798) ccw projected
  arc A67 (-123.4947, 88.4249) -> (-122.7169, 89.6627) centre (-148.5, 105) ccw projected
  arc A68 (-122.7169, 89.6627) -> (-124.0985, 91.5741) centre (-132.9148, 83.7465) ccw projected
  arc A69 (-124.0985, 91.5741) -> (-124.9766, 92.4056) centre (-129.2208, 87.0441) ccw projected
  arc A70 (-124.9766, 92.4056) -> (-125.2845, 92.6173) centre (-126.5375, 90.4655) ccw projected
  line L17 (-126.0004, 92.9992) -> (-125.2845, 92.6173) projected
  arc A71 (-126.0004, 92.9992) -> (-125.0891, 94.8915) centre (-148.5, 105) ccw projected
  line L18 (-124.3442, 94.5699) -> (-125.0891, 94.8915) projected
  arc A72 (-124.3442, 94.5699) -> (-123.9867, 94.4612) centre (-123.4431, 96.8911) ccw projected
  arc A73 (-123.9867, 94.4612) -> (-122.7891, 94.2931) centre (-122.4411, 101.1222) ccw projected
  arc A74 (-122.7891, 94.2931) -> (-120.4333, 94.4046) centre (-122.1661, 106.0664) ccw projected
  arc A75 (-120.4333, 94.4046) -> (-119.9505, 95.7845) centre (-148.5, 105) ccw projected
  arc A76 (-119.9505, 95.7845) -> (-121.7227, 97.3405) centre (-128.5762, 87.7474) ccw projected
  arc A77 (-121.7227, 97.3405) -> (-122.7638, 97.9558) centre (-125.7086, 91.7843) ccw projected
  arc A78 (-122.7638, 97.9558) -> (-123.1112, 98.0937) centre (-123.8539, 95.717) ccw projected
  line L19 (-123.8941, 98.3067) -> (-123.1112, 98.0937) projected
  arc A79 (-123.8941, 98.3067) -> (-123.4267, 100.3544) centre (-148.5, 105) ccw projected
  line L20 (-122.6289, 100.2066) -> (-123.4267, 100.3544) projected
  arc A80 (-122.6289, 100.2066) -> (-122.2561, 100.1801) centre (-122.2669, 102.6701) ccw projected
  arc A81 (-122.2561, 100.1801) -> (-121.0512, 100.2827) centre (-122.2316, 107.0181) ccw projected
  arc A82 (-121.0512, 100.2827) -> (-118.7793, 100.9157) centre (-123.0637, 111.8995) ccw projected
  arc A83 (-118.7793, 100.9157) -> (-118.6156, 102.3684) centre (-148.5, 105) ccw projected
  arc A84 (-118.6156, 102.3684) -> (-120.6897, 103.4911) centre (-125.2367, 92.6134) ccw projected
  arc A85 (-120.6897, 103.4911) -> (-121.8416, 103.8592) centre (-123.3392, 97.1872) ccw projected
  arc A86 (-121.8416, 103.8592) -> (-122.2109, 103.9164) centre (-122.4062, 101.4341) ccw projected
  line L21 (-123.0216, 103.9498) -> (-122.2109, 103.9164) projected
  arc A87 (-123.0216, 103.9498) -> (-123.0216, 106.0502) centre (-148.5, 105) ccw projected
  line L22 (-122.2109, 106.0836) -> (-123.0216, 106.0502) projected
  arc A88 (-122.2109, 106.0836) -> (-121.8416, 106.1408) centre (-122.4062, 108.5659) ccw projected
  arc A89 (-121.8416, 106.1408) -> (-120.6897, 106.5089) centre (-123.3392, 112.8128) ccw projected
  arc A90 (-120.6897, 106.5089) -> (-118.6156, 107.6316) centre (-125.2367, 117.3866) ccw projected
  arc A91 (-118.6156, 107.6316) -> (-118.7793, 109.0843) centre (-148.5, 105) ccw projected
  arc A92 (-118.7793, 109.0843) -> (-121.0512, 109.7173) centre (-123.0637, 98.1005) ccw projected
  arc A93 (-121.0512, 109.7173) -> (-122.2561, 109.8199) centre (-122.2316, 102.9819) ccw projected
  arc A94 (-122.2561, 109.8199) -> (-122.6289, 109.7934) centre (-122.2669, 107.3299) ccw projected
  line L23 (-123.4267, 109.6456) -> (-122.6289, 109.7934) projected
  arc A95 (-123.4267, 109.6456) -> (-123.8941, 111.6933) centre (-148.5, 105) ccw projected
  line L24 (-123.1112, 111.9063) -> (-123.8941, 111.6933) projected
  arc A96 (-123.1112, 111.9063) -> (-122.7638, 112.0442) centre (-123.8539, 114.283) ccw projected
  arc A97 (-122.7638, 112.0442) -> (-121.7227, 112.6595) centre (-125.7086, 118.2157) ccw projected
  arc A98 (-121.7227, 112.6595) -> (-119.9505, 114.2155) centre (-128.5762, 122.2526) ccw projected
  arc A99 (-119.9505, 114.2155) -> (-120.4333, 115.5954) centre (-148.5, 105) ccw projected
  arc A100 (-120.4333, 115.5954) -> (-122.7891, 115.7069) centre (-122.1661, 103.9336) ccw projected
  arc A101 (-122.7891, 115.7069) -> (-123.9867, 115.5388) centre (-122.4411, 108.8778) ccw projected
  arc A102 (-123.9867, 115.5388) -> (-124.3442, 115.4301) centre (-123.4431, 113.1089) ccw projected
  line L25 (-125.0891, 115.1085) -> (-124.3442, 115.4301) projected
  arc A103 (-125.0891, 115.1085) -> (-126.0004, 117.0008) centre (-148.5, 105) ccw projected
  line L26 (-125.2845, 117.3827) -> (-126.0004, 117.0008) projected
  arc A104 (-125.2845, 117.3827) -> (-124.9766, 117.5944) centre (-126.5375, 119.5345) ccw projected
  arc A105 (-124.9766, 117.5944) -> (-124.0985, 118.4259) centre (-129.2208, 122.9559) ccw projected
  arc A106 (-124.0985, 118.4259) -> (-122.7169, 120.3373) centre (-132.9148, 126.2535) ccw projected
  arc A107 (-122.7169, 120.3373) -> (-123.4947, 121.5751) centre (-148.5, 105) ccw projected
  arc A108 (-123.4947, 121.5751) -> (-125.8162, 121.1597) centre (-122.5891, 109.8202) ccw projected
  arc A109 (-125.8162, 121.1597) -> (-126.9464, 120.7293) centre (-123.9573, 114.5792) ccw projected
  arc A110 (-126.9464, 120.7293) -> (-127.2708, 120.5438) centre (-125.8757, 118.4813) ccw projected
  line L27 (-127.9254, 120.0644) -> (-127.2708, 120.5438) projected
  arc A111 (-127.9254, 120.0644) -> (-129.235, 121.7066) centre (-148.5, 105) ccw projected
  line L28 (-128.622, 122.2382) -> (-129.235, 121.7066) projected
  arc A112 (-128.622, 122.2382) -> (-128.3689, 122.5131) centre (-130.3224, 124.0572) ccw projected
  arc A113 (-128.3689, 122.5131) -> (-127.6978, 123.5192) centre (-133.6997, 126.7958) ccw projected
  arc A114 (-127.6978, 123.5192) -> (-126.7762, 125.69) centre (-138.0349, 129.1887) ccw projected
  arc A115 (-126.7762, 125.69) -> (-127.81, 126.7238) centre (-148.5, 105) ccw projected
  arc A116 (-127.81, 126.7238) -> (-129.9808, 125.8022) centre (-124.3113, 115.4651) ccw projected
  arc A117 (-129.9808, 125.8022) -> (-130.9869, 125.1311) centre (-126.7042, 119.8003) ccw projected
  arc A118 (-130.9869, 125.1311) -> (-131.2618, 124.878) centre (-129.4428, 123.1776) ccw projected
  line L29 (-131.7934, 124.265) -> (-131.2618, 124.878) projected
  arc A119 (-131.7934, 124.265) -> (-133.4356, 125.5746) centre (-148.5, 105) ccw projected
  line L30 (-132.9562, 126.2292) -> (-133.4356, 125.5746) projected
  arc A120 (-132.9562, 126.2292) -> (-132.7707, 126.5536) centre (-135.0187, 127.6243) ccw projected
  arc A121 (-132.7707, 126.5536) -> (-132.3403, 127.6838) centre (-138.9208, 129.5427) ccw projected
  arc A122 (-132.3403, 127.6838) -> (-131.9249, 130.0053) centre (-143.6798, 130.9109) ccw projected
  arc A123 (-131.9249, 130.0053) -> (-133.1627, 130.7831) centre (-148.5, 105) ccw projected
  arc A124 (-133.1627, 130.7831) -> (-135.0741, 129.4015) centre (-127.2465, 120.5852) ccw projected
  arc A125 (-135.0741, 129.4015) -> (-135.9056, 128.5234) centre (-130.5441, 124.2792) ccw projected
  arc A126 (-135.9056, 128.5234) -> (-136.1173, 128.2155) centre (-133.9655, 126.9625) ccw projected
  line L31 (-136.4992, 127.4996) -> (-136.1173, 128.2155) projected
  arc A127 (-136.4992, 127.4996) -> (-138.3915, 128.4109) centre (-148.5, 105) ccw projected
  line L32 (-138.0699, 129.1558) -> (-138.3915, 128.4109) projected
  arc A128 (-138.0699, 129.1558) -> (-137.9612, 129.5133) centre (-140.3911, 130.0569) ccw projected
  arc A129 (-137.9612, 129.5133) -> (-137.7931, 130.7109) centre (-144.6222, 131.0589) ccw projected
  arc A130 (-137.7931, 130.7109) -> (-137.9046, 133.0667) centre (-149.5664, 131.3339) ccw projected
  arc A131 (-137.9046, 133.0667) -> (-139.2845, 133.5495) centre (-148.5, 105) ccw projected
  arc A132 (-139.2845, 133.5495) -> (-140.8405, 131.7773) centre (-131.2474, 124.9238) ccw projected
  arc A133 (-140.8405, 131.7773) -> (-141.4558, 130.7362) centre (-135.2843, 127.7914) ccw projected
  arc A134 (-141.4558, 130.7362) -> (-141.5937, 130.3888) centre (-139.217, 129.6461) ccw projected
  line L33 (-141.8067, 129.6059) -> (-141.5937, 130.3888) projected
  arc A135 (-141.8067, 129.6059) -> (-143.8544, 130.0733) centre (-148.5, 105) ccw projected
  line L34 (-143.7066, 130.8711) -> (-143.8544, 130.0733) projected
  arc A136 (-143.7066, 130.8711) -> (-143.6801, 131.2439) centre (-146.1701, 131.2331) ccw projected
  arc A137 (-143.6801, 131.2439) -> (-143.7827, 132.4488) centre (-150.5181, 131.2684) ccw projected
  arc A138 (-143.7827, 132.4488) -> (-144.4157, 134.7207) centre (-155.3995, 130.4363) ccw projected
  arc A139 (-144.4157, 134.7207) -> (-145.8684, 134.8844) centre (-148.5, 105) ccw projected
  arc A140 (-145.8684, 134.8844) -> (-146.9911, 132.8103) centre (-136.1134, 128.2633) ccw projected
  arc A141 (-146.9911, 132.8103) -> (-147.3592, 131.6584) centre (-140.6872, 130.1608) ccw projected
  arc A142 (-147.3592, 131.6584) -> (-147.4164, 131.2891) centre (-144.9341, 131.0938) ccw projected
  line L35 (-147.4498, 130.4784) -> (-147.4164, 131.2891) projected
  arc A143 (-147.4498, 130.4784) -> (-149.5502, 130.4784) centre (-148.5, 105) ccw projected
  line L36 (-149.5836, 131.2891) -> (-149.5502, 130.4784) projected
  arc A144 (-149.5836, 131.2891) -> (-149.6408, 131.6584) centre (-152.0659, 131.0938) ccw projected
  arc A145 (-149.6408, 131.6584) -> (-150.0089, 132.8103) centre (-156.3128, 130.1608) ccw projected
  arc A146 (-150.0089, 132.8103) -> (-151.1316, 134.8844) centre (-160.8866, 128.2633) ccw projected
  arc A147 (-151.1316, 134.8844) -> (-152.5843, 134.7207) centre (-148.5, 105) ccw projected
  arc A148 (-152.5843, 134.7207) -> (-153.2173, 132.4488) centre (-141.6005, 130.4363) ccw projected
  arc A149 (-153.2173, 132.4488) -> (-153.3199, 131.2439) centre (-146.4819, 131.2684) ccw projected
  arc A150 (-153.3199, 131.2439) -> (-153.2934, 130.8711) centre (-150.8299, 131.2331) ccw projected
  line L37 (-153.1456, 130.0733) -> (-153.2934, 130.8711) projected
  arc A151 (-153.1456, 130.0733) -> (-155.1933, 129.6059) centre (-148.5, 105) ccw projected
  line L38 (-155.4063, 130.3888) -> (-155.1933, 129.6059) projected
  arc A152 (-155.4063, 130.3888) -> (-155.5442, 130.7362) centre (-157.783, 129.6461) ccw projected
  arc A153 (-155.5442, 130.7362) -> (-156.1595, 131.7773) centre (-161.7157, 127.7914) ccw projected
  arc A154 (-156.1595, 131.7773) -> (-157.7155, 133.5495) centre (-165.7526, 124.9238) ccw projected
  arc A155 (-157.7155, 133.5495) -> (-159.0954, 133.0667) centre (-148.5, 105) ccw projected
  arc A156 (-159.0954, 133.0667) -> (-159.2069, 130.7109) centre (-147.4336, 131.3339) ccw projected
  arc A157 (-159.2069, 130.7109) -> (-159.0388, 129.5133) centre (-152.3778, 131.0589) ccw projected
  arc A158 (-159.0388, 129.5133) -> (-158.9301, 129.1558) centre (-156.6089, 130.0569) ccw projected
  line L39 (-158.6085, 128.4109) -> (-158.9301, 129.1558) projected
  arc A159 (-158.6085, 128.4109) -> (-160.5008, 127.4996) centre (-148.5, 105) ccw projected
  line L40 (-160.8827, 128.2155) -> (-160.5008, 127.4996) projected
  arc A160 (-160.8827, 128.2155) -> (-161.0944, 128.5234) centre (-163.0345, 126.9625) ccw projected
  arc A161 (-161.0944, 128.5234) -> (-161.9259, 129.4015) centre (-166.4559, 124.2792) ccw projected
  arc A162 (-161.9259, 129.4015) -> (-163.8373, 130.7831) centre (-169.7535, 120.5852) ccw projected
  arc A163 (-163.8373, 130.7831) -> (-165.0751, 130.0053) centre (-148.5, 105) ccw projected
  arc A164 (-165.0751, 130.0053) -> (-164.6597, 127.6838) centre (-153.3202, 130.9109) ccw projected
  arc A165 (-164.6597, 127.6838) -> (-164.2293, 126.5536) centre (-158.0792, 129.5427) ccw projected
  arc A166 (-164.2293, 126.5536) -> (-164.0438, 126.2292) centre (-161.9813, 127.6243) ccw projected
  line L41 (-163.5644, 125.5746) -> (-164.0438, 126.2292) projected
  arc A167 (-163.5644, 125.5746) -> (-165.2066, 124.265) centre (-148.5, 105) ccw projected
  line L42 (-165.7382, 124.878) -> (-165.2066, 124.265) projected
  arc A168 (-165.7382, 124.878) -> (-166.0131, 125.1311) centre (-167.5572, 123.1776) ccw projected
  arc A169 (-166.0131, 125.1311) -> (-167.0192, 125.8022) centre (-170.2958, 119.8003) ccw projected
  arc A170 (-167.0192, 125.8022) -> (-169.19, 126.7238) centre (-172.6887, 115.4651) ccw projected
  arc A171 (-169.19, 126.7238) -> (-170.2238, 125.69) centre (-148.5, 105) ccw projected
  arc A172 (-170.2238, 125.69) -> (-169.3022, 123.5192) centre (-158.9651, 129.1887) ccw projected
  arc A173 (-169.3022, 123.5192) -> (-168.6311, 122.5131) centre (-163.3003, 126.7958) ccw projected
  arc A174 (-168.6311, 122.5131) -> (-168.378, 122.2382) centre (-166.6776, 124.0572) ccw projected
  line L43 (-167.765, 121.7066) -> (-168.378, 122.2382) projected
  arc A175 (-167.765, 121.7066) -> (-169.0746, 120.0644) centre (-148.5, 105) ccw projected
  line L44 (-169.7292, 120.5438) -> (-169.0746, 120.0644) projected
  arc A176 (-169.7292, 120.5438) -> (-170.0536, 120.7293) centre (-171.1243, 118.4813) ccw projected
  arc A177 (-170.0536, 120.7293) -> (-171.1838, 121.1597) centre (-173.0427, 114.5792) ccw projected
  arc A178 (-171.1838, 121.1597) -> (-173.5053, 121.5751) centre (-174.4109, 109.8202) ccw projected
  arc A179 (-173.5053, 121.5751) -> (-174.2831, 120.3373) centre (-148.5, 105) ccw projected
  arc A180 (-174.2831, 120.3373) -> (-172.9015, 118.4259) centre (-164.0852, 126.2535) ccw projected
  arc A181 (-172.9015, 118.4259) -> (-172.0234, 117.5944) centre (-167.7792, 122.9559) ccw projected
  arc A182 (-172.0234, 117.5944) -> (-171.7155, 117.3827) centre (-170.4625, 119.5345) ccw projected
  line L45 (-170.9996, 117.0008) -> (-171.7155, 117.3827) projected
  arc A183 (-170.9996, 117.0008) -> (-171.9109, 115.1085) centre (-148.5, 105) ccw projected
  line L46 (-172.6558, 115.4301) -> (-171.9109, 115.1085) projected
  arc A184 (-172.6558, 115.4301) -> (-173.0133, 115.5388) centre (-173.5569, 113.1089) ccw projected
  arc A185 (-173.0133, 115.5388) -> (-174.2109, 115.7069) centre (-174.5589, 108.8778) ccw projected
  arc A186 (-174.2109, 115.7069) -> (-176.5667, 115.5954) centre (-174.8339, 103.9336) ccw projected
  arc A187 (-176.5667, 115.5954) -> (-177.0495, 114.2155) centre (-148.5, 105) ccw projected
  arc A188 (-177.0495, 114.2155) -> (-175.2773, 112.6595) centre (-168.4238, 122.2526) ccw projected
  arc A189 (-175.2773, 112.6595) -> (-174.2362, 112.0442) centre (-171.2914, 118.2157) ccw projected
  arc A190 (-174.2362, 112.0442) -> (-173.8888, 111.9063) centre (-173.1461, 114.283) ccw projected
  line L47 (-173.1059, 111.6933) -> (-173.8888, 111.9063) projected
  arc A191 (-173.1059, 111.6933) -> (-173.5733, 109.6456) centre (-148.5, 105) ccw projected
  line L48 (-174.3711, 109.7934) -> (-173.5733, 109.6456) projected
  arc A192 (-174.3711, 109.7934) -> (-174.7439, 109.8199) centre (-174.7331, 107.3299) ccw projected
  arc A193 (-174.7439, 109.8199) -> (-175.9488, 109.7173) centre (-174.7684, 102.9819) ccw projected
  arc A194 (-175.9488, 109.7173) -> (-178.2207, 109.0843) centre (-173.9363, 98.1005) ccw projected
  arc A195 (-178.2207, 109.0843) -> (-178.3844, 107.6316) centre (-148.5, 105) ccw projected
  arc A196 (-178.3844, 107.6316) -> (-176.3103, 106.5089) centre (-171.7633, 117.3866) ccw projected
  arc A197 (-176.3103, 106.5089) -> (-175.1584, 106.1408) centre (-173.6608, 112.8128) ccw projected
  arc A198 (-175.1584, 106.1408) -> (-174.7891, 106.0836) centre (-174.5938, 108.5659) ccw projected
  line L49 (-173.9784, 106.0502) -> (-174.7891, 106.0836) projected
  arc A199 (-173.9784, 106.0502) -> (-173.9784, 103.9498) centre (-148.5, 105) ccw projected
  line L50 (-174.7891, 103.9164) -> (-173.9784, 103.9498) projected
  arc A200 (-174.7891, 103.9164) -> (-175.1584, 103.8592) centre (-174.5938, 101.4341) ccw projected
  arc A201 (-175.1584, 103.8592) -> (-176.3103, 103.4911) centre (-173.6608, 97.1872) ccw projected
  arc A202 (-176.3103, 103.4911) -> (-178.3844, 102.3684) centre (-171.7633, 92.6134) ccw projected
  arc A203 (-178.3844, 102.3684) -> (-178.2207, 100.9157) centre (-148.5, 105) ccw projected
  arc A204 (-178.2207, 100.9157) -> (-175.9488, 100.2827) centre (-173.9363, 111.8995) ccw projected
  arc A205 (-175.9488, 100.2827) -> (-174.7439, 100.1801) centre (-174.7684, 107.0181) ccw projected
  arc A206 (-174.7439, 100.1801) -> (-174.3711, 100.2066) centre (-174.7331, 102.6701) ccw projected
  line L51 (-173.5733, 100.3544) -> (-174.3711, 100.2066) projected
  arc A207 (-173.5733, 100.3544) -> (-173.1059, 98.3067) centre (-148.5, 105) ccw projected
  line L52 (-173.8888, 98.0937) -> (-173.1059, 98.3067) projected
  arc A208 (-173.8888, 98.0937) -> (-174.2362, 97.9558) centre (-173.1461, 95.717) ccw projected
  arc A209 (-174.2362, 97.9558) -> (-175.2773, 97.3405) centre (-171.2914, 91.7843) ccw projected
  arc A210 (-175.2773, 97.3405) -> (-177.0495, 95.7845) centre (-168.4238, 87.7474) ccw projected
  arc A211 (-177.0495, 95.7845) -> (-176.5667, 94.4046) centre (-148.5, 105) ccw projected
  arc A212 (-176.5667, 94.4046) -> (-174.2109, 94.2931) centre (-174.8339, 106.0664) ccw projected
  arc A213 (-174.2109, 94.2931) -> (-173.0133, 94.4612) centre (-174.5589, 101.1222) ccw projected
  arc A214 (-173.0133, 94.4612) -> (-172.6558, 94.5699) centre (-173.5569, 96.8911) ccw projected
  line L53 (-171.9109, 94.8915) -> (-172.6558, 94.5699) projected
  arc A215 (-171.9109, 94.8915) -> (-170.9996, 92.9992) centre (-148.5, 105) ccw projected
  line L54 (-171.7155, 92.6173) -> (-170.9996, 92.9992) projected
  arc A216 (-171.7155, 92.6173) -> (-172.0234, 92.4056) centre (-170.4625, 90.4655) ccw projected
  arc A217 (-172.0234, 92.4056) -> (-172.9015, 91.5741) centre (-167.7792, 87.0441) ccw projected
  arc A218 (-172.9015, 91.5741) -> (-174.2831, 89.6627) centre (-164.0852, 83.7465) ccw projected
  arc A219 (-174.2831, 89.6627) -> (-173.5053, 88.4249) centre (-148.5, 105) ccw projected
  arc A220 (-173.5053, 88.4249) -> (-171.1838, 88.8403) centre (-174.4109, 100.1798) ccw projected
  arc A221 (-171.1838, 88.8403) -> (-170.0536, 89.2707) centre (-173.0427, 95.4208) ccw projected
  arc A222 (-170.0536, 89.2707) -> (-169.7292, 89.4562) centre (-171.1243, 91.5187) ccw projected
  line L55 (-169.0746, 89.9356) -> (-169.7292, 89.4562) projected
  arc A223 (-169.0746, 89.9356) -> (-167.765, 88.2934) centre (-148.5, 105) ccw projected
  arc A224 (-147.3388, 98.1857) -> (-148.5, 98.8449) centre (-148.8502, 96.8758) ccw projected
  line L56 (-138.2915, 87.7462) -> (-147.3388, 98.1857) projected
  arc A225 (-138.9544, 84.6252) -> (-138.2915, 87.7462) centre (-139.8029, 86.4363) ccw projected
  arc A226 (-158.0456, 84.6252) -> (-138.9544, 84.6252) centre (-148.5, 105) ccw projected
  arc A227 (-158.7085, 87.7462) -> (-158.0456, 84.6252) centre (-157.1971, 86.4363) ccw projected
  line L57 (-149.6612, 98.1857) -> (-158.7085, 87.7462) projected
  arc A228 (-148.5, 98.8449) -> (-149.6612, 98.1857) centre (-148.1498, 96.8758) ccw projected
  arc A229 (-148.5, 98.8449) -> (-148.7641, 98.874) centre (-148.8502, 96.8758) ccw projected
  arc A230 (-148.7641, 98.874) -> (-148.2359, 98.874) centre (-148.5, 105) ccw projected
  arc A231 (-148.2359, 98.874) -> (-148.5, 98.8449) centre (-148.1498, 96.8758) ccw projected
  arc A232 (-154.622, 101.7899) -> (-154.3538, 103.098) centre (-156.3348, 102.8226) ccw projected
  line L58 (-161.7547, 89.9594) -> (-154.622, 101.7899) projected
  arc A233 (-164.9278, 89.6254) -> (-161.7547, 89.9594) centre (-163.4675, 90.992) ccw projected
  arc A234 (-170.8273, 107.7823) -> (-164.9278, 89.6254) centre (-148.5, 105) ccw projected
  arc A235 (-168.064, 109.3772) -> (-170.8273, 107.7823) centre (-168.8427, 107.535) ccw projected
  line L59 (-155.3396, 103.9986) -> (-168.064, 109.3772) projected
  arc A236 (-154.3538, 103.098) -> (-155.3396, 103.9986) centre (-156.1183, 102.1564) ccw projected
  arc A237 (-154.3538, 103.098) -> (-154.4078, 103.3581) centre (-156.3348, 102.8226) ccw projected
  arc A238 (-154.4078, 103.3581) -> (-154.2446, 102.8558) centre (-148.5, 105) ccw projected
  arc A239 (-154.2446, 102.8558) -> (-154.3538, 103.098) centre (-156.1183, 102.1564) ccw projected
  arc A240 (-142.6462, 103.098) -> (-142.7554, 102.8558) centre (-140.8817, 102.1564) ccw projected
  arc A241 (-142.7554, 102.8558) -> (-142.5922, 103.3581) centre (-148.5, 105) ccw projected